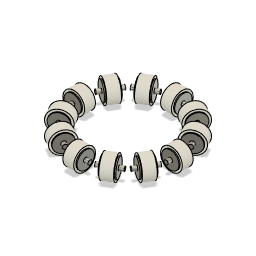
サイドホイール (Autodesk Fusion 360 design; units mm, degrees)
Autodesk Fusion 360 part; units mm, degrees
(part 1 of 3)
sketch "スケッチ1" plane through (0, 0.2306, 0) normal (0, 1, 0) x (-1, 0, 0)
  circle A0 centre (0.8985, -52.106) radius 15.5
  circle A1 centre (-6.9391, -68.3808) radius 1.5
  circle A2 centre (15.0212, -40.8435) radius 1.5
  circle A3 centre (-16.7123, -56.1256) radius 1.5
  circle A4 centre (8.736, -68.3808) radius 1.5
  circle A5 centre (0.8985, -34.0424) radius 1.5
  circle A6 centre (-13.2243, -40.8435) radius 1.5
  circle A7 centre (18.5092, -56.1256) radius 1.5
  arc A8 (-27.629, -49.2874) -> (-27.8547, -48.9282) centre (-27.9215, -49.2206) ccw
  line L0 (-27.8547, -48.9282) -> (-28.4097, -48.8015)
  arc A9 (-28.4097, -48.8015) -> (-28.9994, -49.6325) centre (-28.0028, -49.7149) ccw
  arc A10 (-28.9994, -49.6325) -> (-28.9994, -54.5796) centre (0.8985, -52.106) ccw
  arc A11 (-28.9994, -54.5796) -> (-28.4097, -55.4106) centre (-28.0028, -54.4971) ccw
  line L1 (-28.4097, -55.4106) -> (-27.8547, -55.2839)
  arc A12 (-27.8547, -55.2839) -> (-27.629, -54.9246) centre (-27.9215, -54.9914) ccw
  line L2 (-27.629, -54.9246) -> (-27.8404, -53.9985)
  arc A13 (-27.088, -52.801) -> (-27.8404, -53.9985) centre (-26.8654, -53.7759) ccw
  line L3 (-27.088, -52.801) -> (-26.308, -52.623)
  arc A14 (-25.1106, -53.3754) -> (-26.308, -52.623) centre (-26.0855, -53.5979) ccw
  line L4 (-25.1106, -53.3754) -> (-24.8992, -54.3016)
  arc A15 (-24.8992, -54.3016) -> (-24.5399, -54.5273) centre (-24.6067, -54.2348) ccw
  line L5 (-24.5399, -54.5273) -> (-20.6402, -53.6372)
  arc A16 (-19.4428, -54.3896) -> (-20.6402, -53.6372) centre (-20.4177, -54.6122) ccw
  line L6 (-19.4428, -54.3896) -> (-18.4192, -58.8743)
  arc A17 (-19.1716, -60.0718) -> (-18.4192, -58.8743) centre (-19.3941, -59.0968) ccw
  line L7 (-19.1716, -60.0718) -> (-22.9738, -60.9396)
  arc A18 (-22.9738, -60.9396) -> (-23.1995, -61.2988) centre (-22.9071, -61.2321) ccw
  line L8 (-23.1995, -61.2988) -> (-22.9881, -62.225)
  arc A19 (-23.7405, -63.4224) -> (-22.9881, -62.225) centre (-23.9631, -62.4475) ccw
  line L9 (-23.7405, -63.4224) -> (-24.618, -63.6227)
  arc A20 (-25.8154, -62.8703) -> (-24.618, -63.6227) centre (-24.8405, -62.6478) ccw
  line L10 (-25.8154, -62.8703) -> (-26.0268, -61.9441)
  arc A21 (-26.0268, -61.9441) -> (-26.3861, -61.7184) centre (-26.3193, -62.0109) ccw
  line L11 (-26.3861, -61.7184) -> (-26.9411, -61.8451)
  arc A22 (-26.9411, -61.8451) -> (-27.1118, -62.8496) centre (-26.1781, -62.4915) ccw
  arc A23 (-27.1118, -62.8496) -> (-24.9653, -67.3068) centre (0.8985, -52.106) ccw
  arc A24 (-24.9653, -67.3068) -> (-24.0735, -67.7997) centre (-24.1032, -66.8001) ccw
  line L12 (-24.0735, -67.7997) -> (-23.6284, -67.4447)
  arc A25 (-23.6284, -67.4447) -> (-23.5809, -67.0231) centre (-23.8155, -67.2102) ccw
  line L13 (-23.5809, -67.0231) -> (-24.1732, -66.2804)
  arc A26 (-24.0149, -64.8751) -> (-24.1732, -66.2804) centre (-23.3914, -65.6569) ccw
  line L14 (-24.0149, -64.8751) -> (-23.3894, -64.3763)
  arc A27 (-21.9841, -64.5346) -> (-23.3894, -64.3763) centre (-22.7659, -65.1581) ccw
  line L15 (-21.9841, -64.5346) -> (-21.3918, -65.2773)
  arc A28 (-21.3918, -65.2773) -> (-20.9702, -65.3248) centre (-21.1572, -65.0903) ccw
  line L16 (-20.9702, -65.3248) -> (-17.8429, -62.8309)
  arc A29 (-16.4375, -62.9892) -> (-17.8429, -62.8309) centre (-17.2194, -63.6127) ccw
  line L17 (-16.4375, -62.9892) -> (-13.5695, -66.5856)
  arc A30 (-13.7278, -67.991) -> (-13.5695, -66.5856) centre (-14.3513, -67.2091) ccw
  line L18 (-13.7278, -67.991) -> (-16.777, -70.4226)
  arc A31 (-16.777, -70.4226) -> (-16.8245, -70.8442) centre (-16.5899, -70.6571) ccw
  line L19 (-16.8245, -70.8442) -> (-16.2322, -71.5869)
  arc A32 (-16.3905, -72.9922) -> (-16.2322, -71.5869) centre (-17.014, -72.2104) ccw
  line L20 (-16.3905, -72.9922) -> (-17.0942, -73.5534)
  arc A33 (-18.4995, -73.395) -> (-17.0942, -73.5534) centre (-17.7176, -72.7715) ccw
  line L21 (-18.4995, -73.395) -> (-19.0918, -72.6523)
  arc A34 (-19.0918, -72.6523) -> (-19.5134, -72.6048) centre (-19.3263, -72.8393) ccw
  line L22 (-19.5134, -72.6048) -> (-19.9585, -72.9598)
  arc A35 (-19.9585, -72.9598) -> (-19.6764, -73.9389) centre (-18.9906, -73.2111) ccw
  arc A36 (-19.6764, -73.9389) -> (-15.8087, -77.0233) centre (0.8985, -52.106) ccw
  arc A37 (-15.8087, -77.0233) -> (-14.7913, -77.0804) centre (-15.2517, -76.1928) ccw
  line L23 (-14.7913, -77.0804) -> (-14.5443, -76.5675)
  arc A38 (-14.5443, -76.5675) -> (-14.6844, -76.1671) centre (-14.8146, -76.4374) ccw
  line L24 (-14.6844, -76.1671) -> (-15.5403, -75.7549)
  arc A39 (-16.0074, -74.42) -> (-15.5403, -75.7549) centre (-15.1065, -74.8539) ccw
  line L25 (-16.0074, -74.42) -> (-15.6603, -73.6992)
  arc A40 (-14.3255, -73.2322) -> (-15.6603, -73.6992) centre (-14.7593, -74.1331) ccw
  line L26 (-14.3255, -73.2322) -> (-13.4695, -73.6443)
  arc A41 (-13.4695, -73.6443) -> (-13.0691, -73.5042) centre (-13.3394, -73.3741) ccw
  line L27 (-13.0691, -73.5042) -> (-11.3335, -69.9003)
  arc A42 (-9.9987, -69.4333) -> (-11.3335, -69.9003) centre (-10.4326, -70.3342) ccw
  line L28 (-9.9987, -69.4333) -> (-5.8542, -71.4291)
  arc A43 (-5.3872, -72.764) -> (-5.8542, -71.4291) centre (-6.2881, -72.3301) ccw
  line L29 (-5.3872, -72.764) -> (-7.0793, -76.2778)
  arc A44 (-7.0793, -76.2778) -> (-6.9392, -76.6782) centre (-6.809, -76.4079) ccw
  line L30 (-6.9392, -76.6782) -> (-6.0833, -77.0904)
  arc A45 (-5.6162, -78.4253) -> (-6.0833, -77.0904) centre (-6.5171, -77.9914) ccw
  line L31 (-5.6162, -78.4253) -> (-6.0067, -79.2361)
  arc A46 (-7.3415, -79.7032) -> (-6.0067, -79.2361) centre (-6.9076, -78.8022) ccw
  line L32 (-7.3415, -79.7032) -> (-8.1974, -79.291)
  arc A47 (-8.1974, -79.291) -> (-8.5979, -79.4312) centre (-8.3276, -79.5613) ccw
  line L33 (-8.5979, -79.4312) -> (-8.8449, -79.9441)
  arc A48 (-8.8449, -79.9441) -> (-8.1659, -80.7039) centre (-7.8638, -79.7506) ccw
  arc A49 (-8.1659, -80.7039) -> (-3.3429, -81.8047) centre (0.8985, -52.106) ccw
  arc A50 (-3.3429, -81.8047) -> (-2.4015, -81.4147) centre (-3.2015, -80.8147) ccw
  line L34 (-2.4015, -81.4147) -> (-2.4015, -80.8454)
  arc A51 (-2.4015, -80.8454) -> (-2.7015, -80.5454) centre (-2.7015, -80.8454) ccw
  line L35 (-2.7015, -80.5454) -> (-3.6515, -80.5454)
  arc A52 (-4.6515, -79.5454) -> (-3.6515, -80.5454) centre (-3.6515, -79.5454) ccw
  line L36 (-4.6515, -79.5454) -> (-4.6515, -78.7454)
  arc A53 (-3.6515, -77.7454) -> (-4.6515, -78.7454) centre (-3.6515, -78.7454) ccw
  line L37 (-3.6515, -77.7454) -> (-2.7015, -77.7454)
  arc A54 (-2.7015, -77.7454) -> (-2.4015, -77.4454) centre (-2.7015, -77.4454) ccw
  line L38 (-2.4015, -77.4454) -> (-2.4015, -73.4454)
  arc A55 (-1.4015, -72.4454) -> (-2.4015, -73.4454) centre (-1.4015, -73.4454) ccw
  line L39 (-1.4015, -72.4454) -> (3.1985, -72.4454)
  arc A56 (4.1985, -73.4454) -> (3.1985, -72.4454) centre (3.1985, -73.4454) ccw
  line L40 (4.1985, -73.4454) -> (4.1985, -77.3454)
  arc A57 (4.1985, -77.3454) -> (4.4985, -77.6454) centre (4.4985, -77.3454) ccw
  line L41 (4.4985, -77.6454) -> (5.4485, -77.6454)
  arc A58 (6.4485, -78.6454) -> (5.4485, -77.6454) centre (5.4485, -78.6454) ccw
  line L42 (6.4485, -78.6454) -> (6.4485, -79.5454)
  arc A59 (5.4485, -80.5454) -> (6.4485, -79.5454) centre (5.4485, -79.5454) ccw
  line L43 (5.4485, -80.5454) -> (4.4985, -80.5454)
  arc A60 (4.4985, -80.5454) -> (4.1985, -80.8454) centre (4.4985, -80.8454) ccw
  line L44 (4.1985, -80.8454) -> (4.1985, -81.4147)
  arc A61 (4.1985, -81.4147) -> (5.1398, -81.8047) centre (4.9985, -80.8147) ccw
  arc A62 (5.1398, -81.8047) -> (9.9629, -80.7039) centre (0.8985, -52.106) ccw
  arc A63 (9.9629, -80.7039) -> (10.6418, -79.9441) centre (9.6607, -79.7506) ccw
  line L45 (10.6418, -79.9441) -> (10.3948, -79.4312)
  arc A64 (10.3948, -79.4312) -> (9.9944, -79.291) centre (10.1245, -79.5613) ccw
  line L46 (9.9944, -79.291) -> (9.1385, -79.7032)
  arc A65 (7.8036, -79.2361) -> (9.1385, -79.7032) centre (8.7046, -78.8022) ccw
  line L47 (7.8036, -79.2361) -> (7.4565, -78.5154)
  arc A66 (7.9236, -77.1805) -> (7.4565, -78.5154) centre (8.3575, -78.0815) ccw
  line L48 (7.9236, -77.1805) -> (8.7795, -76.7683)
  arc A67 (8.7795, -76.7683) -> (8.9196, -76.3679) centre (8.6493, -76.498) ccw
  line L49 (8.9196, -76.3679) -> (7.1841, -72.764)
  arc A68 (7.6512, -71.4291) -> (7.1841, -72.764) centre (8.0851, -72.3301) ccw
  line L50 (7.6512, -71.4291) -> (11.7956, -69.4333)
  arc A69 (13.1305, -69.9003) -> (11.7956, -69.4333) centre (12.2295, -70.3342) ccw
  line L51 (13.1305, -69.9003) -> (14.8226, -73.4141)
  arc A70 (14.8226, -73.4141) -> (15.2231, -73.5543) centre (15.0929, -73.284) ccw
  line L52 (15.2231, -73.5543) -> (16.079, -73.1421)
  arc A71 (17.4139, -73.6091) -> (16.079, -73.1421) centre (16.5129, -74.043) ccw
  line L53 (17.4139, -73.6091) -> (17.8044, -74.42)
  arc A72 (17.3373, -75.7549) -> (17.8044, -74.42) centre (16.9034, -74.8539) ccw
  line L54 (17.3373, -75.7549) -> (16.4814, -76.1671)
  arc A73 (16.4814, -76.1671) -> (16.3412, -76.5675) centre (16.6115, -76.4374) ccw
  line L55 (16.3412, -76.5675) -> (16.5882, -77.0804)
  arc A74 (16.5882, -77.0804) -> (17.6056, -77.0233) centre (17.0487, -76.1928) ccw
  arc A75 (17.6056, -77.0233) -> (21.3207, -74.0818) centre (0.8985, -52.106) ccw
  arc A76 (21.3207, -74.0818) -> (21.3281, -72.6237) centre (20.6399, -73.3492) ccw
  arc A77 (21.3281, -72.6237) -> (20.8871, -72.6543) centre (21.1217, -72.8414) ccw
  line L56 (20.8871, -72.6543) -> (20.2964, -73.395)
  arc A78 (18.8911, -73.5534) -> (20.2964, -73.395) centre (19.5146, -72.7715) ccw
  line L57 (18.8911, -73.5534) -> (18.2656, -73.0546)
  arc A79 (18.1073, -71.6493) -> (18.2656, -73.0546) centre (18.8891, -72.2728) ccw
  line L58 (18.1073, -71.6493) -> (18.6996, -70.9065)
  arc A80 (18.6996, -70.9065) -> (18.6521, -70.4849) centre (18.465, -70.7195) ccw
  line L59 (18.6521, -70.4849) -> (15.5248, -67.991)
  arc A81 (15.3664, -66.5856) -> (15.5248, -67.991) centre (16.1483, -67.2091) ccw
  line L60 (15.3664, -66.5856) -> (18.2345, -62.9892)
  arc A82 (19.6398, -62.8309) -> (18.2345, -62.9892) centre (19.0163, -63.6127) ccw
  line L61 (19.6398, -62.8309) -> (22.6889, -65.2625)
  arc A83 (22.6889, -65.2625) -> (23.1105, -65.215) centre (22.876, -65.0279) ccw
  line L62 (23.1105, -65.215) -> (23.7029, -64.4723)
  arc A84 (25.1082, -64.3139) -> (23.7029, -64.4723) centre (24.4847, -65.0957) ccw
  line L63 (25.1082, -64.3139) -> (25.8118, -64.8751)
  arc A85 (25.9702, -66.2804) -> (25.8118, -64.8751) centre (25.1883, -65.6569) ccw
  line L64 (25.9702, -66.2804) -> (25.3795, -67.0211)
  arc A86 (25.3795, -67.0211) -> (25.4477, -67.4579) centre (25.614, -67.2081) ccw
  arc A87 (25.4477, -67.4579) -> (26.8676, -67.1262) centre (26.002, -66.6255) ccw
  arc A88 (26.8676, -67.1262) -> (28.9087, -62.8496) centre (0.8985, -52.106) ccw
  arc A89 (28.9087, -62.8496) -> (28.738, -61.8451) centre (27.9751, -62.4915) ccw
  line L65 (28.738, -61.8451) -> (28.183, -61.7184)
  arc A90 (28.183, -61.7184) -> (27.8238, -61.9441) centre (28.1162, -62.0109) ccw
  line L66 (27.8238, -61.9441) -> (27.6124, -62.8703)
  arc A91 (26.4149, -63.6227) -> (27.6124, -62.8703) centre (26.6374, -62.6478) ccw
  line L67 (26.4149, -63.6227) -> (25.635, -63.4447)
  arc A92 (24.8826, -62.2473) -> (25.635, -63.4447) centre (25.8575, -62.4698) ccw
  line L68 (24.8826, -62.2473) -> (25.094, -61.3211)
  arc A93 (25.094, -61.3211) -> (24.8682, -60.9618) centre (24.8015, -61.2543) ccw
  line L69 (24.8682, -60.9618) -> (20.9685, -60.0718)
  arc A94 (20.2161, -58.8743) -> (20.9685, -60.0718) centre (21.1911, -59.0968) ccw
  line L70 (20.2161, -58.8743) -> (21.2397, -54.3896)
  arc A95 (22.4372, -53.6372) -> (21.2397, -54.3896) centre (22.2146, -54.6122) ccw
  line L71 (22.4372, -53.6372) -> (26.2394, -54.5051)
  arc A96 (26.2394, -54.5051) -> (26.5986, -54.2793) centre (26.3061, -54.2126) ccw
  line L72 (26.5986, -54.2793) -> (26.81, -53.3532)
  arc A97 (28.0075, -52.6007) -> (26.81, -53.3532) centre (27.7849, -53.5757) ccw
  line L73 (28.0075, -52.6007) -> (28.8849, -52.801)
  arc A98 (29.6373, -53.9985) -> (28.8849, -52.801) centre (28.6624, -53.7759) ccw
  line L74 (29.6373, -53.9985) -> (29.4259, -54.9246)
  arc A99 (29.4259, -54.9246) -> (29.6516, -55.2839) centre (29.7184, -54.9914) ccw
  line L75 (29.6516, -55.2839) -> (30.2067, -55.4106)
  arc A100 (30.2067, -55.4106) -> (30.7963, -54.5796) centre (29.7997, -54.4971) ccw
  arc A101 (30.7963, -54.5796) -> (30.7963, -49.6325) centre (0.8985, -52.106) ccw
  arc A102 (30.7963, -49.6325) -> (30.2067, -48.8015) centre (29.7997, -49.7149) ccw
  line L76 (30.2067, -48.8015) -> (29.6516, -48.9282)
  arc A103 (29.6516, -48.9282) -> (29.4259, -49.2874) centre (29.7184, -49.2206) ccw
  line L77 (29.4259, -49.2874) -> (29.6373, -50.2136)
  arc A104 (28.8849, -51.411) -> (29.6373, -50.2136) centre (28.6624, -50.4361) ccw
  line L78 (28.8849, -51.411) -> (28.105, -51.5891)
  arc A105 (26.9075, -50.8366) -> (28.105, -51.5891) centre (27.8824, -50.6141) ccw
  line L79 (26.9075, -50.8366) -> (26.6961, -49.9105)
  arc A106 (26.6961, -49.9105) -> (26.3369, -49.6847) centre (26.4036, -49.9772) ccw
  line L80 (26.3369, -49.6847) -> (22.4372, -50.5748)
  arc A107 (21.2397, -49.8224) -> (22.4372, -50.5748) centre (22.2146, -49.5999) ccw
  line L81 (21.2397, -49.8224) -> (20.2161, -45.3377)
  arc A108 (20.9685, -44.1403) -> (20.2161, -45.3377) centre (21.1911, -45.1152) ccw
  line L82 (20.9685, -44.1403) -> (24.7707, -43.2725)
  arc A109 (24.7707, -43.2725) -> (24.9965, -42.9132) centre (24.704, -42.98) ccw
  line L83 (24.9965, -42.9132) -> (24.7851, -41.9871)
  arc A110 (25.5375, -40.7896) -> (24.7851, -41.9871) centre (25.76, -41.7645) ccw
  line L84 (25.5375, -40.7896) -> (26.4149, -40.5893)
  arc A111 (27.6124, -41.3417) -> (26.4149, -40.5893) centre (26.6374, -41.5643) ccw
  line L85 (27.6124, -41.3417) -> (27.8238, -42.2679)
  arc A112 (27.8238, -42.2679) -> (28.183, -42.4936) centre (28.1162, -42.2012) ccw
  line L86 (28.183, -42.4936) -> (28.738, -42.367)
  arc A113 (28.738, -42.367) -> (28.9087, -41.3624) centre (27.9751, -41.7205) ccw
  arc A114 (28.9087, -41.3624) -> (26.7623, -36.9053) centre (0.8985, -52.106) ccw
  arc A115 (26.7623, -36.9053) -> (25.8705, -36.4124) centre (25.9001, -37.4119) ccw
  line L87 (25.8705, -36.4124) -> (25.4254, -36.7673)
  arc A116 (25.4254, -36.7673) -> (25.3779, -37.1889) centre (25.6124, -37.0019) ccw
  line L88 (25.3779, -37.1889) -> (25.9702, -37.9317)
  arc A117 (25.8118, -39.337) -> (25.9702, -37.9317) centre (25.1883, -38.5552) ccw
  line L89 (25.8118, -39.337) -> (25.1864, -39.8358)
  arc A118 (23.781, -39.6775) -> (25.1864, -39.8358) centre (24.5629, -39.054) ccw
  line L90 (23.781, -39.6775) -> (23.1887, -38.9347)
  arc A119 (23.1887, -38.9347) -> (22.7671, -38.8872) centre (22.9542, -39.1218) ccw
  line L91 (22.7671, -38.8872) -> (19.6398, -41.3812)
  arc A120 (18.2345, -41.2228) -> (19.6398, -41.3812) centre (19.0163, -40.5993) ccw
  line L92 (18.2345, -41.2228) -> (15.3664, -37.6264)
  arc A121 (15.5248, -36.2211) -> (15.3664, -37.6264) centre (16.1483, -37.0029) ccw
  line L93 (15.5248, -36.2211) -> (18.5739, -33.7895)
  arc A122 (18.5739, -33.7895) -> (18.6214, -33.3679) centre (18.3869, -33.5549) ccw
  line L94 (18.6214, -33.3679) -> (18.0291, -32.6251)
  arc A123 (18.1874, -31.2198) -> (18.0291, -32.6251) centre (18.8109, -32.0016) ccw
  line L95 (18.1874, -31.2198) -> (18.8911, -30.6587)
  arc A124 (20.2964, -30.817) -> (18.8911, -30.6587) centre (19.5146, -31.4405) ccw
  line L96 (20.2964, -30.817) -> (20.8887, -31.5598)
  arc A125 (20.8887, -31.5598) -> (21.3103, -31.6073) centre (21.1233, -31.3727) ccw
  line L97 (21.3103, -31.6073) -> (21.7554, -31.2523)
  arc A126 (21.7554, -31.2523) -> (21.4734, -30.2732) centre (20.7875, -31.0009) ccw
  arc A127 (21.4734, -30.2732) -> (17.6056, -27.1887) centre (0.8985, -52.106) ccw
  arc A128 (17.6056, -27.1887) -> (16.5882, -27.1316) centre (17.0487, -28.0193) ccw
  line L98 (16.5882, -27.1316) -> (16.3412, -27.6445)
  arc A129 (16.3412, -27.6445) -> (16.4814, -28.045) centre (16.6115, -27.7747) ccw
  line L99 (16.4814, -28.045) -> (17.3373, -28.4572)
  arc A130 (17.8044, -29.792) -> (17.3373, -28.4572) centre (16.9034, -29.3581) ccw
  line L100 (17.8044, -29.792) -> (17.4572, -30.5128)
  arc A131 (16.1224, -30.9799) -> (17.4572, -30.5128) centre (16.5563, -30.0789) ccw
  line L101 (16.1224, -30.9799) -> (15.2665, -30.5677)
  arc A132 (15.2665, -30.5677) -> (14.866, -30.7078) centre (15.1363, -30.838) ccw
  line L102 (14.866, -30.7078) -> (13.1305, -34.3117)
  arc A133 (11.7956, -34.7788) -> (13.1305, -34.3117) centre (12.2295, -33.8778) ccw
  line L103 (11.7956, -34.7788) -> (7.6512, -32.7829)
  arc A134 (7.1841, -31.4481) -> (7.6512, -32.7829) centre (8.0851, -31.882) ccw
  line L104 (7.1841, -31.4481) -> (8.8762, -27.9343)
  arc A135 (8.8762, -27.9343) -> (8.7361, -27.5338) centre (8.6059, -27.8041) ccw
  line L105 (8.7361, -27.5338) -> (7.8802, -27.1216)
  arc A136 (7.4131, -25.7868) -> (7.8802, -27.1216) centre (8.3141, -26.2207) ccw
  line L106 (7.4131, -25.7868) -> (7.8036, -24.9759)
  arc A137 (9.1385, -24.5088) -> (7.8036, -24.9759) centre (8.7046, -25.4098) ccw
  line L107 (9.1385, -24.5088) -> (9.9944, -24.921)
  arc A138 (9.9944, -24.921) -> (10.3948, -24.7809) centre (10.1245, -24.6507) ccw
  line L108 (10.3948, -24.7809) -> (10.6418, -24.268)
  arc A139 (10.6418, -24.268) -> (9.9629, -23.5082) centre (9.6607, -24.4614) ccw
  arc A140 (9.9629, -23.5082) -> (5.1398, -22.4074) centre (0.8985, -52.106) ccw
  arc A141 (5.1398, -22.4074) -> (4.1985, -22.7973) centre (4.9985, -23.3973) ccw
  line L109 (4.1985, -22.7973) -> (4.1985, -23.3666)
  arc A142 (4.1985, -23.3666) -> (4.4985, -23.6666) centre (4.4985, -23.3666) ccw
  line L110 (4.4985, -23.6666) -> (5.4485, -23.6666)
  arc A143 (6.4485, -24.6666) -> (5.4485, -23.6666) centre (5.4485, -24.6666) ccw
  line L111 (6.4485, -24.6666) -> (6.4485, -25.4666)
  arc A144 (5.4485, -26.4666) -> (6.4485, -25.4666) centre (5.4485, -25.4666) ccw
  line L112 (5.4485, -26.4666) -> (4.4985, -26.4666)
  arc A145 (4.4985, -26.4666) -> (4.1985, -26.7666) centre (4.4985, -26.7666) ccw
  line L113 (4.1985, -26.7666) -> (4.1985, -30.7666)
  arc A146 (3.1985, -31.7666) -> (4.1985, -30.7666) centre (3.1985, -30.7666) ccw
  line L114 (3.1985, -31.7666) -> (-1.4015, -31.7666)
  arc A147 (-2.4015, -30.7666) -> (-1.4015, -31.7666) centre (-1.4015, -30.7666) ccw
  line L115 (-2.4015, -30.7666) -> (-2.4015, -26.8666)
  arc A148 (-2.4015, -26.8666) -> (-2.7015, -26.5666) centre (-2.7015, -26.8666) ccw
  line L116 (-2.7015, -26.5666) -> (-3.6515, -26.5666)
  arc A149 (-4.6515, -25.5666) -> (-3.6515, -26.5666) centre (-3.6515, -25.5666) ccw
  line L117 (-4.6515, -25.5666) -> (-4.6515, -24.6666)
  arc A150 (-3.6515, -23.6666) -> (-4.6515, -24.6666) centre (-3.6515, -24.6666) ccw
  line L118 (-3.6515, -23.6666) -> (-2.7015, -23.6666)
  arc A151 (-2.7015, -23.6666) -> (-2.4015, -23.3666) centre (-2.7015, -23.3666) ccw
  line L119 (-2.4015, -23.3666) -> (-2.4015, -22.7973)
  arc A152 (-2.4015, -22.7973) -> (-3.3429, -22.4074) centre (-3.2015, -23.3973) ccw
  arc A153 (-3.3429, -22.4074) -> (-8.1659, -23.5082) centre (0.8985, -52.106) ccw
  arc A154 (-8.1659, -23.5082) -> (-8.8449, -24.268) centre (-7.8638, -24.4614) ccw
  line L120 (-8.8449, -24.268) -> (-8.5979, -24.7809)
  arc A155 (-8.5979, -24.7809) -> (-8.1974, -24.921) centre (-8.3276, -24.6507) ccw
  line L121 (-8.1974, -24.921) -> (-7.3415, -24.5088)
  arc A156 (-6.0067, -24.9759) -> (-7.3415, -24.5088) centre (-6.9076, -25.4098) ccw
  line L122 (-6.0067, -24.9759) -> (-5.6596, -25.6967)
  arc A157 (-6.1266, -27.0316) -> (-5.6596, -25.6967) centre (-6.5605, -26.1306) ccw
  line L123 (-6.1266, -27.0316) -> (-6.9826, -27.4437)
  arc A158 (-6.9826, -27.4437) -> (-7.1227, -27.8442) centre (-6.8524, -27.714) ccw
  line L124 (-7.1227, -27.8442) -> (-5.3872, -31.4481)
  arc A159 (-5.8542, -32.7829) -> (-5.3872, -31.4481) centre (-6.2881, -31.882) ccw
  line L125 (-5.8542, -32.7829) -> (-9.9987, -34.7788)
  arc A160 (-11.3335, -34.3117) -> (-9.9987, -34.7788) centre (-10.4326, -33.8778) ccw
  line L126 (-11.3335, -34.3117) -> (-13.0257, -30.7979)
  arc A161 (-13.0257, -30.7979) -> (-13.4262, -30.6578) centre (-13.296, -30.9281) ccw
  line L127 (-13.4262, -30.6578) -> (-14.2821, -31.07)
  arc A162 (-15.6169, -30.6029) -> (-14.2821, -31.07) centre (-14.716, -30.169) ccw
  line L128 (-15.6169, -30.6029) -> (-16.0074, -29.792)
  arc A163 (-15.5403, -28.4572) -> (-16.0074, -29.792) centre (-15.1065, -29.3581) ccw
  line L129 (-15.5403, -28.4572) -> (-14.6844, -28.045)
  arc A164 (-14.6844, -28.045) -> (-14.5443, -27.6445) centre (-14.8146, -27.7747) ccw
  line L130 (-14.5443, -27.6445) -> (-14.7913, -27.1316)
  arc A165 (-14.7913, -27.1316) -> (-15.8087, -27.1887) centre (-15.2517, -28.0193) ccw
  arc A166 (-15.8087, -27.1887) -> (-19.6764, -30.2732) centre (0.8985, -52.106) ccw
  arc A167 (-19.6764, -30.2732) -> (-19.9585, -31.2523) centre (-18.9906, -31.0009) ccw
  line L131 (-19.9585, -31.2523) -> (-19.5134, -31.6073)
  arc A168 (-19.5134, -31.6073) -> (-19.0918, -31.5598) centre (-19.3263, -31.3727) ccw
  line L132 (-19.0918, -31.5598) -> (-18.4995, -30.817)
  arc A169 (-17.0942, -30.6587) -> (-18.4995, -30.817) centre (-17.7176, -31.4405) ccw
  line L133 (-17.0942, -30.6587) -> (-16.4687, -31.1575)
  arc A170 (-16.3103, -32.5628) -> (-16.4687, -31.1575) centre (-17.0922, -31.9393) ccw
  line L134 (-16.3103, -32.5628) -> (-16.9027, -33.3055)
  arc A171 (-16.9027, -33.3055) -> (-16.8552, -33.7271) centre (-16.6681, -33.4926) ccw
  line L135 (-16.8552, -33.7271) -> (-13.7278, -36.2211)
  arc A172 (-13.5695, -37.6264) -> (-13.7278, -36.2211) centre (-14.3513, -37.0029) ccw
  line L136 (-13.5695, -37.6264) -> (-16.4375, -41.2228)
  arc A173 (-17.8429, -41.3812) -> (-16.4375, -41.2228) centre (-17.2194, -40.5993) ccw
  line L137 (-17.8429, -41.3812) -> (-20.892, -38.9496)
  arc A174 (-20.892, -38.9496) -> (-21.3136, -38.9971) centre (-21.0791, -39.1841) ccw
  line L138 (-21.3136, -38.9971) -> (-21.9059, -39.7398)
  arc A175 (-23.3112, -39.8981) -> (-21.9059, -39.7398) centre (-22.6878, -39.1163) ccw
  line L139 (-23.3112, -39.8981) -> (-24.0149, -39.337)
  arc A176 (-24.1732, -37.9317) -> (-24.0149, -39.337) centre (-23.3914, -38.5552) ccw
  line L140 (-24.1732, -37.9317) -> (-23.5809, -37.1889)
  arc A177 (-23.5809, -37.1889) -> (-23.6284, -36.7673) centre (-23.8155, -37.0019) ccw
  line L141 (-23.6284, -36.7673) -> (-24.0735, -36.4124)
  arc A178 (-24.0735, -36.4124) -> (-24.9653, -36.9053) centre (-24.1032, -37.4119) ccw
  arc A179 (-24.9653, -36.9053) -> (-27.1118, -41.3624) centre (0.8985, -52.106) ccw
  arc A180 (-27.1118, -41.3624) -> (-26.9411, -42.367) centre (-26.1781, -41.7205) ccw
  line L142 (-26.9411, -42.367) -> (-26.3861, -42.4936)
  arc A181 (-26.3861, -42.4936) -> (-26.0268, -42.2679) centre (-26.3193, -42.2012) ccw
  line L143 (-26.0268, -42.2679) -> (-25.8154, -41.3417)
  arc A182 (-24.618, -40.5893) -> (-25.8154, -41.3417) centre (-24.8405, -41.5643) ccw
  line L144 (-24.618, -40.5893) -> (-23.838, -40.7674)
  arc A183 (-23.0856, -41.9648) -> (-23.838, -40.7674) centre (-24.0606, -41.7423) ccw
  line L145 (-23.0856, -41.9648) -> (-23.297, -42.891)
  arc A184 (-23.297, -42.891) -> (-23.0713, -43.2502) centre (-23.0045, -42.9577) ccw
  line L146 (-23.0713, -43.2502) -> (-19.1716, -44.1403)
  arc A185 (-18.4192, -45.3377) -> (-19.1716, -44.1403) centre (-19.3941, -45.1152) ccw
  line L147 (-18.4192, -45.3377) -> (-19.4428, -49.8224)
  arc A186 (-20.6402, -50.5748) -> (-19.4428, -49.8224) centre (-20.4177, -49.5999) ccw
  line L148 (-20.6402, -50.5748) -> (-24.4424, -49.707)
  arc A187 (-24.4424, -49.707) -> (-24.8017, -49.9327) centre (-24.5092, -49.9995) ccw
  line L149 (-24.8017, -49.9327) -> (-25.0131, -50.8589)
  arc A188 (-26.2105, -51.6113) -> (-25.0131, -50.8589) centre (-25.988, -50.6364) ccw
  line L150 (-26.2105, -51.6113) -> (-27.088, -51.411)
  arc A189 (-27.8404, -50.2136) -> (-27.088, -51.411) centre (-26.8654, -50.4361) ccw
  line L151 (-27.8404, -50.2136) -> (-27.629, -49.2874)
  line L152 (4.1985, -80.8454) -> (4.1985, -80.8)
  line L153 (4.1985, -81.4147) -> (4.1985, -81.9391)
  line L154 (-2.4015, -81.4147) -> (-2.4015, -81.9846)
  line L155 (4.1985, -81.4147) -> (4.1985, -80.5454)
  line L156 (4.4985, -80.5454) -> (4.1985, -80.5454)
  line L157 (4.4985, -80.5454) -> (6.4485, -80.5454)
  line L158 (6.4485, -79.5454) -> (6.4485, -80.5454)
  line L159 (6.4485, -79.5454) -> (6.4485, -77.6454)
  line L160 (5.4485, -77.6454) -> (6.4485, -77.6454)
  line L161 (5.4485, -77.6454) -> (4.1985, -77.6454)
  line L162 (4.1985, -77.3454) -> (4.1985, -77.6454)
  line L163 (4.1985, -77.3454) -> (4.1985, -72.4454)
  line L164 (3.1985, -72.4454) -> (4.1985, -72.4454)
  line L165 (3.1985, -72.4454) -> (-2.4015, -72.4454)
  line L166 (-2.4015, -73.4454) -> (-2.4015, -72.4454)
  line L167 (-2.4015, -73.4454) -> (-2.4015, -77.7454)
  line L168 (-3.1765, -77.7454) -> (-2.4015, -77.7454)
  line L169 (-3.1765, -77.7454) -> (-4.6515, -77.7454)
  line L170 (-4.6515, -78.7454) -> (-4.6515, -77.7454)
  line L171 (-4.6515, -78.7454) -> (-4.6515, -80.5454)
  line L172 (-3.6515, -80.5454) -> (-4.6515, -80.5454)
  line L173 (-3.6515, -80.5454) -> (-2.4015, -80.5454)
  line L174 (-2.4015, -81.4147) -> (-2.4015, -80.5454)
  line L175 (5.55, -232.8464) -> (5.55, -231.9464)
  line L176 (3.6, -233.8464) -> (4.55, -233.8464)
  line L177 (-3.6, -233.8464) -> (-4.55, -233.8464)
  line L178 (-5.55, -232.0464) -> (-5.55, -232.8464)
  line L179 (-3.3, -234.1464) -> (-3.3, -234.7095)
  line L180 (-3.3, -226.7464) -> (-3.3, -230.7464)
  line L181 (3.3, -234.1464) -> (3.3, -234.7095)
  line L182 (-3.6, -231.0464) -> (-4.55, -231.0464)
  line L183 (4.55, -230.9464) -> (3.6, -230.9464)
  line L184 (2.3, -225.7464) -> (-2.3, -225.7464)
  line L185 (3.3, -230.6464) -> (3.3, -226.7464)
  arc A190 (4.55, -233.8464) -> (5.55, -232.8464) centre (4.55, -232.8464) ccw
  arc A191 (5.55, -231.9464) -> (4.55, -230.9464) centre (4.55, -231.9464) ccw
  arc A192 (-5.55, -232.8464) -> (-4.55, -233.8464) centre (-4.55, -232.8464) ccw
  arc A193 (-4.55, -231.0464) -> (-5.55, -232.0464) centre (-4.55, -232.0464) ccw
  arc A194 (3.3, -226.7464) -> (2.3, -225.7464) centre (2.3, -226.7464) ccw
  arc A195 (-2.3, -225.7464) -> (-3.3, -226.7464) centre (-2.3, -226.7464) ccw
  arc A196 (3.3, -230.6464) -> (3.6, -230.9464) centre (3.6, -230.6464) ccw
  arc A197 (3.6, -233.8464) -> (3.3, -234.1464) centre (3.6, -234.1464) ccw
  arc A198 (-3.3, -234.1464) -> (-3.6, -233.8464) centre (-3.6, -234.1464) ccw
  arc A199 (-3.6, -231.0464) -> (-3.3, -230.7464) centre (-3.6, -230.7464) ccw
  arc A200 (3.3, -234.7095) -> (3.876, -235.2037) centre (3.8, -234.7095) ccw
  arc A201 (-3.876, -235.2037) -> (-3.3, -234.7095) centre (-3.8, -234.7095) ccw
  arc A202 (9.2153, -232.5614) -> (8.8055, -232.4516) centre (8.9555, -232.7114) ccw
  arc A203 (6.5828, -230.5018) -> (6.2168, -231.8678) centre (7.0828, -231.3678) ccw
  arc A204 (5.8814, -224.7868) -> (5.5153, -226.1528) centre (6.3814, -225.6528) ccw
  arc A205 (11.2311, -222.8528) -> (9.8651, -222.4868) centre (10.3651, -223.3528) ccw
  line L186 (14.9311, -229.2614) -> (15.2126, -229.7491)
  line L187 (8.8055, -232.4516) -> (7.9828, -232.9266)
  arc A206 (9.2451, -233.765) -> (9.4969, -233.0491) centre (9.0639, -233.2991) ccw
  line L188 (6.2168, -231.8678) -> (6.6168, -232.5606)
  line L189 (7.4055, -230.0268) -> (6.5828, -230.5018)
  line L190 (9.2153, -232.5614) -> (9.4969, -233.0491)
  line L191 (13.1811, -226.2303) -> (11.2311, -222.8528)
  arc A207 (6.6168, -232.5606) -> (7.9828, -232.9266) centre (7.4828, -232.0606) ccw
  line L192 (9.8651, -222.4868) -> (5.8814, -224.7868)
  arc A208 (7.4055, -230.0268) -> (7.5153, -229.6169) centre (7.2555, -229.7669) ccw
  line L193 (5.5153, -226.1528) -> (7.5153, -229.6169)
  arc A209 (15.2126, -229.7491) -> (15.9586, -229.889) centre (15.6457, -229.4991) ccw
  arc A210 (15.7797, -226.2312) -> (14.4136, -225.8651) centre (14.9136, -226.7312) ccw
  line L194 (15.0409, -228.8516) -> (15.8636, -228.3766)
  line L195 (16.2297, -227.0106) -> (15.7797, -226.2312)
  line L196 (14.4136, -225.8651) -> (13.5909, -226.3401)
  arc A211 (15.0409, -228.8516) -> (14.9311, -229.2614) centre (15.1909, -229.1114) ccw
  arc A212 (13.1811, -226.2303) -> (13.5909, -226.3401) centre (13.4409, -226.0803) ccw
  arc A213 (15.8636, -228.3766) -> (16.2297, -227.0106) centre (15.3636, -227.5106) ccw
  arc A214 (19.2614, -224.9311) -> (18.8516, -225.0409) centre (19.1114, -225.1909) ccw
  arc A215 (15.9517, -224.4636) -> (16.3178, -225.8297) centre (16.8178, -224.9636) ccw
  arc A216 (12.4868, -219.8651) -> (12.8528, -221.2311) centre (13.3528, -220.3651) ccw
  arc A217 (16.1528, -215.5153) -> (14.7868, -215.8814) centre (15.6528, -216.3814) ccw
  line L197 (22.5614, -219.2153) -> (23.0491, -219.4969)
  line L198 (18.8516, -225.0409) -> (18.3766, -225.8636)
  arc A218 (19.889, -225.9586) -> (19.7491, -225.2126) centre (19.4991, -225.6457) ccw
  line L199 (16.3178, -225.8297) -> (17.0106, -226.2297)
  line L200 (16.4267, -223.6409) -> (15.9517, -224.4636)
  line L201 (19.2614, -224.9311) -> (19.7491, -225.2126)
  line L202 (19.5303, -217.4653) -> (16.1528, -215.5153)
  arc A219 (17.0106, -226.2297) -> (18.3766, -225.8636) centre (17.5106, -225.3636) ccw
  line L203 (14.7868, -215.8814) -> (12.4868, -219.8651)
  arc A220 (16.4267, -223.6409) -> (16.3169, -223.2311) centre (16.1669, -223.4909) ccw
  line L204 (12.8528, -221.2311) -> (16.3169, -223.2311)
  arc A221 (23.0491, -219.4969) -> (23.765, -219.2451) centre (23.2991, -219.0639) ccw
  arc A222 (21.7812, -216.1668) -> (20.4151, -216.5328) centre (21.2812, -217.0328) ccw
  line L205 (22.4516, -218.8055) -> (22.9266, -217.9828)
  line L206 (22.5606, -216.6168) -> (21.7812, -216.1668)
  line L207 (20.4151, -216.5328) -> (19.9401, -217.3555)
  arc A223 (22.4516, -218.8055) -> (22.5614, -219.2153) centre (22.7114, -218.9555) ccw
  arc A224 (19.5303, -217.4653) -> (19.9401, -217.3555) centre (19.6803, -217.2055) ccw
  arc A225 (22.9266, -217.9828) -> (22.5606, -216.6168) centre (22.0606, -217.4828) ccw
  arc A226 (24.1464, -213.3) -> (23.8464, -213.6) centre (24.1464, -213.6) ccw
  arc A227 (21.0464, -214.55) -> (22.0464, -215.55) centre (22.0464, -214.55) ccw
  arc A228 (15.7464, -212.3) -> (16.7464, -213.3) centre (16.7464, -212.3) ccw
  arc A229 (16.7464, -206.7) -> (15.7464, -207.7) centre (16.7464, -207.7) ccw
  line L208 (24.1464, -206.7) -> (24.7095, -206.7)
  line L209 (23.8464, -213.6) -> (23.8464, -214.55)
  arc A230 (25.2037, -213.876) -> (24.7095, -213.3) centre (24.7095, -213.8) ccw
  line L210 (22.0464, -215.55) -> (22.8464, -215.55)
  line L211 (21.0464, -213.6) -> (21.0464, -214.55)
  line L212 (24.1464, -213.3) -> (24.7095, -213.3)
  line L213 (20.6464, -206.7) -> (16.7464, -206.7)
  arc A231 (22.8464, -215.55) -> (23.8464, -214.55) centre (22.8464, -214.55) ccw
  line L214 (15.7464, -207.7) -> (15.7464, -212.3)
  arc A232 (21.0464, -213.6) -> (20.7464, -213.3) centre (20.7464, -213.6) ccw
  line L215 (16.7464, -213.3) -> (20.7464, -213.3)
  arc A233 (24.7095, -206.7) -> (25.2037, -206.124) centre (24.7095, -206.2) ccw
  arc A234 (21.9464, -204.45) -> (20.9464, -205.45) centre (21.9464, -205.45) ccw
  line L216 (23.8464, -206.4) -> (23.8464, -205.45)
  line L217 (22.8464, -204.45) -> (21.9464, -204.45)
  line L218 (20.9464, -205.45) -> (20.9464, -206.4)
  arc A235 (23.8464, -206.4) -> (24.1464, -206.7) centre (24.1464, -206.4) ccw
  arc A236 (20.6464, -206.7) -> (20.9464, -206.4) centre (20.6464, -206.4) ccw
  arc A237 (23.8464, -205.45) -> (22.8464, -204.45) centre (22.8464, -205.45) ccw
  arc A238 (22.5614, -200.7847) -> (22.4516, -201.1945) centre (22.7114, -201.0445) ccw
  arc A239 (20.5017, -203.4172) -> (21.8678, -203.7832) centre (21.3678, -202.9172) ccw
  arc A240 (14.7868, -204.1186) -> (16.1528, -204.4847) centre (15.6528, -203.6186) ccw
  arc A241 (12.8528, -198.7689) -> (12.4868, -200.1349) centre (13.3528, -199.6349) ccw
  line L219 (19.2614, -195.0689) -> (19.7491, -194.7874)
  line L220 (22.4516, -201.1945) -> (22.9266, -202.0172)
  arc A242 (23.765, -200.7549) -> (23.0491, -200.5031) centre (23.2991, -200.9361) ccw
  line L221 (21.8678, -203.7832) -> (22.5606, -203.3832)
  line L222 (20.0267, -202.5945) -> (20.5017, -203.4172)
  line L223 (22.5614, -200.7847) -> (23.0491, -200.5031)
  line L224 (16.2303, -196.8189) -> (12.8528, -198.7689)
  arc A243 (22.5606, -203.3832) -> (22.9266, -202.0172) centre (22.0606, -202.5172) ccw
  line L225 (12.4868, -200.1349) -> (14.7868, -204.1186)
  arc A244 (20.0267, -202.5945) -> (19.6169, -202.4847) centre (19.7669, -202.7445) ccw
  line L226 (16.1528, -204.4847) -> (19.6169, -202.4847)
  arc A245 (19.7491, -194.7874) -> (19.889, -194.0414) centre (19.4991, -194.3544) ccw
  arc A246 (16.2312, -194.2203) -> (15.8651, -195.5864) centre (16.7312, -195.0864) ccw
  line L227 (18.8516, -194.9591) -> (18.3766, -194.1364)
  line L228 (17.0106, -193.7703) -> (16.2312, -194.2203)
  line L229 (15.8651, -195.5864) -> (16.3401, -196.4091)
  arc A247 (18.8516, -194.9591) -> (19.2614, -195.0689) centre (19.1114, -194.8091) ccw
  arc A248 (16.2303, -196.8189) -> (16.3401, -196.4091) centre (16.0803, -196.5591) ccw
  arc A249 (18.3766, -194.1364) -> (17.0106, -193.7703) centre (17.5106, -194.6364) ccw
  arc A250 (14.9311, -190.7386) -> (15.0409, -191.1484) centre (15.1909, -190.8886) ccw
  arc A251 (14.4636, -194.0483) -> (15.8297, -193.6822) centre (14.9636, -193.1822) ccw
  arc A252 (9.8651, -197.5132) -> (11.2311, -197.1472) centre (10.3651, -196.6472) ccw
  arc A253 (5.5153, -193.8472) -> (5.8814, -195.2132) centre (6.3814, -194.3472) ccw
  line L230 (9.2153, -187.4386) -> (9.4969, -186.9509)
  line L231 (15.0409, -191.1484) -> (15.8636, -191.6234)
  arc A254 (15.9586, -190.111) -> (15.2126, -190.2509) centre (15.6457, -190.5009) ccw
  line L232 (15.8297, -193.6822) -> (16.2297, -192.9894)
  line L233 (13.6409, -193.5733) -> (14.4636, -194.0483)
  line L234 (14.9311, -190.7386) -> (15.2126, -190.2509)
  line L235 (7.4653, -190.4697) -> (5.5153, -193.8472)
  arc A255 (16.2297, -192.9894) -> (15.8636, -191.6234) centre (15.3636, -192.4894) ccw
  line L236 (5.8814, -195.2132) -> (9.8651, -197.5132)
  arc A256 (13.6409, -193.5733) -> (13.2311, -193.6831) centre (13.4909, -193.8331) ccw
  line L237 (11.2311, -197.1472) -> (13.2311, -193.6831)
  arc A257 (9.4969, -186.9509) -> (9.2451, -186.235) centre (9.0639, -186.7009) ccw
  arc A258 (6.1668, -188.2188) -> (6.5328, -189.5849) centre (7.0328, -188.7188) ccw
  line L238 (8.8055, -187.5484) -> (7.9828, -187.0734)
  line L239 (6.6168, -187.4394) -> (6.1668, -188.2188)
  line L240 (6.5328, -189.5849) -> (7.3555, -190.0599)
  arc A259 (8.8055, -187.5484) -> (9.2153, -187.4386) centre (8.9555, -187.2886) ccw
  arc A260 (7.4653, -190.4697) -> (7.3555, -190.0599) centre (7.2055, -190.3197) ccw
  arc A261 (7.9828, -187.0734) -> (6.6168, -187.4394) centre (7.4828, -187.9394) ccw
  arc A262 (3.3, -185.8536) -> (3.6, -186.1536) centre (3.6, -185.8536) ccw
  arc A263 (4.55, -188.9536) -> (5.55, -187.9536) centre (4.55, -187.9536) ccw
  arc A264 (2.3, -194.2536) -> (3.3, -193.2536) centre (2.3, -193.2536) ccw
  arc A265 (-3.3, -193.2536) -> (-2.3, -194.2536) centre (-2.3, -193.2536) ccw
  line L241 (-3.3, -185.8536) -> (-3.3, -185.2905)
  line L242 (3.6, -186.1536) -> (4.55, -186.1536)
  arc A266 (3.876, -184.7963) -> (3.3, -185.2905) centre (3.8, -185.2905) ccw
  line L243 (5.55, -187.9536) -> (5.55, -187.1536)
  line L244 (3.6, -188.9536) -> (4.55, -188.9536)
  line L245 (3.3, -185.8536) -> (3.3, -185.2905)
  line L246 (-3.3, -189.3536) -> (-3.3, -193.2536)
  arc A267 (5.55, -187.1536) -> (4.55, -186.1536) centre (4.55, -187.1536) ccw
  line L247 (-2.3, -194.2536) -> (2.3, -194.2536)
  arc A268 (3.6, -188.9536) -> (3.3, -189.2536) centre (3.6, -189.2536) ccw
  line L248 (3.3, -193.2536) -> (3.3, -189.2536)
  arc A269 (-3.3, -185.2905) -> (-3.876, -184.7963) centre (-3.8, -185.2905) ccw
  arc A270 (-5.55, -188.0536) -> (-4.55, -189.0536) centre (-4.55, -188.0536) ccw
  line L249 (-3.6, -186.1536) -> (-4.55, -186.1536)
  line L250 (-5.55, -187.1536) -> (-5.55, -188.0536)
  line L251 (-4.55, -189.0536) -> (-3.6, -189.0536)
  arc A271 (-3.6, -186.1536) -> (-3.3, -185.8536) centre (-3.6, -185.8536) ccw
  arc A272 (-3.3, -189.3536) -> (-3.6, -189.0536) centre (-3.6, -189.3536) ccw
  arc A273 (-4.55, -186.1536) -> (-5.55, -187.1536) centre (-4.55, -187.1536) ccw
  arc A274 (-9.2153, -187.4386) -> (-8.8055, -187.5484) centre (-8.9555, -187.2886) ccw
  arc A275 (-6.5828, -189.4983) -> (-6.2168, -188.1322) centre (-7.0828, -188.6322) ccw
  arc A276 (-5.8814, -195.2132) -> (-5.5153, -193.8472) centre (-6.3814, -194.3472) ccw
  arc A277 (-11.2311, -197.1472) -> (-9.8651, -197.5132) centre (-10.3651, -196.6472) ccw
  line L252 (-14.9311, -190.7386) -> (-15.2126, -190.2509)
  line L253 (-8.8055, -187.5484) -> (-7.9828, -187.0734)
  arc A278 (-9.2451, -186.235) -> (-9.4969, -186.9509) centre (-9.0639, -186.7009) ccw
  line L254 (-6.2168, -188.1322) -> (-6.6168, -187.4394)
  line L255 (-7.4055, -189.9733) -> (-6.5828, -189.4983)
  line L256 (-9.2153, -187.4386) -> (-9.4969, -186.9509)
  line L257 (-13.1811, -193.7697) -> (-11.2311, -197.1472)
  arc A279 (-6.6168, -187.4394) -> (-7.9828, -187.0734) centre (-7.4828, -187.9394) ccw
  line L258 (-9.8651, -197.5132) -> (-5.8814, -195.2132)
  arc A280 (-7.4055, -189.9733) -> (-7.5153, -190.3831) centre (-7.2555, -190.2331) ccw
  line L259 (-5.5153, -193.8472) -> (-7.5153, -190.3831)
  arc A281 (-15.2126, -190.2509) -> (-15.9586, -190.111) centre (-15.6457, -190.5009) ccw
  arc A282 (-15.7797, -193.7688) -> (-14.4136, -194.1349) centre (-14.9136, -193.2688) ccw
  line L260 (-15.0409, -191.1484) -> (-15.8636, -191.6234)
  line L261 (-16.2297, -192.9894) -> (-15.7797, -193.7688)
  line L262 (-14.4136, -194.1349) -> (-13.5909, -193.6599)
  arc A283 (-15.0409, -191.1484) -> (-14.9311, -190.7386) centre (-15.1909, -190.8886) ccw
  arc A284 (-13.1811, -193.7697) -> (-13.5909, -193.6599) centre (-13.4409, -193.9197) ccw
  arc A285 (-15.8636, -191.6234) -> (-16.2297, -192.9894) centre (-15.3636, -192.4894) ccw
  arc A286 (-19.2614, -195.0689) -> (-18.8516, -194.9591) centre (-19.1114, -194.8091) ccw
  arc A287 (-15.9517, -195.5364) -> (-16.3178, -194.1703) centre (-16.8178, -195.0364) ccw
  arc A288 (-12.4868, -200.1349) -> (-12.8528, -198.7689) centre (-13.3528, -199.6349) ccw
  arc A289 (-16.1528, -204.4847) -> (-14.7868, -204.1186) centre (-15.6528, -203.6186) ccw
  line L263 (-22.5614, -200.7847) -> (-23.0491, -200.5031)
  line L264 (-18.8516, -194.9591) -> (-18.3766, -194.1364)
  arc A290 (-19.889, -194.0414) -> (-19.7491, -194.7874) centre (-19.4991, -194.3544) ccw
  line L265 (-16.3178, -194.1703) -> (-17.0106, -193.7703)
  line L266 (-16.4267, -196.3591) -> (-15.9517, -195.5364)
  line L267 (-19.2614, -195.0689) -> (-19.7491, -194.7874)
  line L268 (-19.5303, -202.5347) -> (-16.1528, -204.4847)
  arc A291 (-17.0106, -193.7703) -> (-18.3766, -194.1364) centre (-17.5106, -194.6364) ccw
  line L269 (-14.7868, -204.1186) -> (-12.4868, -200.1349)
  arc A292 (-16.4267, -196.3591) -> (-16.3169, -196.7689) centre (-16.1669, -196.5091) ccw
  line L270 (-12.8528, -198.7689) -> (-16.3169, -196.7689)
  arc A293 (-23.0491, -200.5031) -> (-23.765, -200.7549) centre (-23.2991, -200.9361) ccw
  arc A294 (-21.7812, -203.8332) -> (-20.4151, -203.4672) centre (-21.2812, -202.9672) ccw
  line L271 (-22.4516, -201.1945) -> (-22.9266, -202.0172)
  line L272 (-22.5606, -203.3832) -> (-21.7812, -203.8332)
  line L273 (-20.4151, -203.4672) -> (-19.9401, -202.6445)
  arc A295 (-22.4516, -201.1945) -> (-22.5614, -200.7847) centre (-22.7114, -201.0445) ccw
  arc A296 (-19.5303, -202.5347) -> (-19.9401, -202.6445) centre (-19.6803, -202.7945) ccw
  arc A297 (-22.9266, -202.0172) -> (-22.5606, -203.3832) centre (-22.0606, -202.5172) ccw
  arc A298 (-24.1464, -206.7) -> (-23.8464, -206.4) centre (-24.1464, -206.4) ccw
  arc A299 (-21.0464, -205.45) -> (-22.0464, -204.45) centre (-22.0464, -205.45) ccw
  arc A300 (-15.7464, -207.7) -> (-16.7464, -206.7) centre (-16.7464, -207.7) ccw
  arc A301 (-16.7464, -213.3) -> (-15.7464, -212.3) centre (-16.7464, -212.3) ccw
  line L274 (-24.1464, -213.3) -> (-24.7095, -213.3)
  line L275 (-23.8464, -206.4) -> (-23.8464, -205.45)
  arc A302 (-25.2037, -206.124) -> (-24.7095, -206.7) centre (-24.7095, -206.2) ccw
  line L276 (-22.0464, -204.45) -> (-22.8464, -204.45)
  line L277 (-21.0464, -206.4) -> (-21.0464, -205.45)
  line L278 (-24.1464, -206.7) -> (-24.7095, -206.7)
  line L279 (-20.6464, -213.3) -> (-16.7464, -213.3)
  arc A303 (-22.8464, -204.45) -> (-23.8464, -205.45) centre (-22.8464, -205.45) ccw
  line L280 (-15.7464, -212.3) -> (-15.7464, -207.7)
  arc A304 (-21.0464, -206.4) -> (-20.7464, -206.7) centre (-20.7464, -206.4) ccw
  line L281 (-16.7464, -206.7) -> (-20.7464, -206.7)
  arc A305 (-24.7095, -213.3) -> (-25.2037, -213.876) centre (-24.7095, -213.8) ccw
  arc A306 (-21.9464, -215.55) -> (-20.9464, -214.55) centre (-21.9464, -214.55) ccw
  line L282 (-23.8464, -213.6) -> (-23.8464, -214.55)
  line L283 (-22.8464, -215.55) -> (-21.9464, -215.55)
  line L284 (-20.9464, -214.55) -> (-20.9464, -213.6)
  arc A307 (-23.8464, -213.6) -> (-24.1464, -213.3) centre (-24.1464, -213.6) ccw
  arc A308 (-20.6464, -213.3) -> (-20.9464, -213.6) centre (-20.6464, -213.6) ccw
  arc A309 (-23.8464, -214.55) -> (-22.8464, -215.55) centre (-22.8464, -214.55) ccw
  arc A310 (-22.5614, -219.2153) -> (-22.4516, -218.8055) centre (-22.7114, -218.9555) ccw
  arc A311 (-20.5017, -216.5828) -> (-21.8678, -216.2168) centre (-21.3678, -217.0828) ccw
  arc A312 (-14.7868, -215.8814) -> (-16.1528, -215.5153) centre (-15.6528, -216.3814) ccw
  arc A313 (-12.8528, -221.2311) -> (-12.4868, -219.8651) centre (-13.3528, -220.3651) ccw
  line L285 (-19.2614, -224.9311) -> (-19.7491, -225.2126)
  line L286 (-22.4516, -218.8055) -> (-22.9266, -217.9828)
  arc A314 (-23.765, -219.2451) -> (-23.0491, -219.4969) centre (-23.2991, -219.0639) ccw
  line L287 (-21.8678, -216.2168) -> (-22.5606, -216.6168)
  line L288 (-20.0267, -217.4055) -> (-20.5017, -216.5828)
  line L289 (-22.5614, -219.2153) -> (-23.0491, -219.4969)
  line L290 (-16.2303, -223.1811) -> (-12.8528, -221.2311)
  arc A315 (-22.5606, -216.6168) -> (-22.9266, -217.9828) centre (-22.0606, -217.4828) ccw
  line L291 (-12.4868, -219.8651) -> (-14.7868, -215.8814)
  arc A316 (-20.0267, -217.4055) -> (-19.6169, -217.5153) centre (-19.7669, -217.2555) ccw
  line L292 (-16.1528, -215.5153) -> (-19.6169, -217.5153)
  arc A317 (-19.7491, -225.2126) -> (-19.889, -225.9586) centre (-19.4991, -225.6457) ccw
  arc A318 (-16.2312, -225.7797) -> (-15.8651, -224.4136) centre (-16.7312, -224.9136) ccw
  line L293 (-18.8516, -225.0409) -> (-18.3766, -225.8636)
  line L294 (-17.0106, -226.2297) -> (-16.2312, -225.7797)
  line L295 (-15.8651, -224.4136) -> (-16.3401, -223.5909)
  arc A319 (-18.8516, -225.0409) -> (-19.2614, -224.9311) centre (-19.1114, -225.1909) ccw
  arc A320 (-16.2303, -223.1811) -> (-16.3401, -223.5909) centre (-16.0803, -223.4409) ccw
  arc A321 (-18.3766, -225.8636) -> (-17.0106, -226.2297) centre (-17.5106, -225.3636) ccw
  arc A322 (-14.9311, -229.2614) -> (-15.0409, -228.8516) centre (-15.1909, -229.1114) ccw
  arc A323 (-14.4636, -225.9518) -> (-15.8297, -226.3178) centre (-14.9636, -226.8178) ccw
  arc A324 (-9.8651, -222.4868) -> (-11.2311, -222.8528) centre (-10.3651, -223.3528) ccw
  arc A325 (-5.5153, -226.1528) -> (-5.8814, -224.7868) centre (-6.3814, -225.6528) ccw
  line L296 (-9.2153, -232.5614) -> (-9.4969, -233.0491)
  line L297 (-15.0409, -228.8516) -> (-15.8636, -228.3766)
  arc A326 (-15.9586, -229.889) -> (-15.2126, -229.7491) centre (-15.6457, -229.4991) ccw
  line L298 (-15.8297, -226.3178) -> (-16.2297, -227.0106)
  line L299 (-13.6409, -226.4268) -> (-14.4636, -225.9518)
  line L300 (-14.9311, -229.2614) -> (-15.2126, -229.7491)
  line L301 (-7.4653, -229.5303) -> (-5.5153, -226.1528)
  arc A327 (-16.2297, -227.0106) -> (-15.8636, -228.3766) centre (-15.3636, -227.5106) ccw
  line L302 (-5.8814, -224.7868) -> (-9.8651, -222.4868)
  arc A328 (-13.6409, -226.4268) -> (-13.2311, -226.3169) centre (-13.4909, -226.1669) ccw
  line L303 (-11.2311, -222.8528) -> (-13.2311, -226.3169)
  arc A329 (-9.4969, -233.0491) -> (-9.2451, -233.765) centre (-9.0639, -233.2991) ccw
  arc A330 (-6.1668, -231.7812) -> (-6.5328, -230.4151) centre (-7.0328, -231.2812) ccw
  line L304 (-8.8055, -232.4516) -> (-7.9828, -232.9266)
  line L305 (-6.6168, -232.5606) -> (-6.1668, -231.7812)
  line L306 (-6.5328, -230.4151) -> (-7.3555, -229.9401)
  arc A331 (-8.8055, -232.4516) -> (-9.2153, -232.5614) centre (-8.9555, -232.7114) ccw
  arc A332 (-7.4653, -229.5303) -> (-7.3555, -229.9401) centre (-7.2055, -229.6803) ccw
  arc A333 (-7.9828, -232.9266) -> (-6.6168, -232.5606) centre (-7.4828, -232.0606) ccw
  arc A334 (3.876, -235.2037) -> (9.2451, -233.765) centre (0, -210) ccw
  arc A335 (15.9586, -229.889) -> (19.889, -225.9586) centre (0, -210) ccw
  arc A336 (23.765, -219.2451) -> (25.2037, -213.876) centre (0, -210) ccw
  arc A337 (25.2037, -206.124) -> (23.765, -200.7549) centre (0, -210) ccw
  arc A338 (19.889, -194.0414) -> (15.9586, -190.111) centre (0, -210) ccw
  arc A339 (9.2451, -186.235) -> (3.876, -184.7963) centre (0, -210) ccw
  arc A340 (-3.876, -184.7963) -> (-9.2451, -186.235) centre (0, -210) ccw
  arc A341 (-15.9586, -190.111) -> (-19.889, -194.0414) centre (0, -210) ccw
  arc A342 (-23.765, -200.7549) -> (-25.2037, -206.124) centre (0, -210) ccw
  arc A343 (-25.2037, -213.876) -> (-23.765, -219.2451) centre (0, -210) ccw
  arc A344 (-19.889, -225.9586) -> (-15.9586, -229.889) centre (0, -210) ccw
  arc A345 (-9.2451, -233.765) -> (-3.876, -235.2037) centre (0, -210) ccw
  line L307 (3.3, -234.1464) -> (3.3, -230.6464)
  line L308 (-3.3, -234.1464) -> (-3.3, -230.7464)
  line L309 (14.9311, -229.2614) -> (13.1811, -226.2303)
  line L310 (9.2153, -232.5614) -> (7.5153, -229.6169)
  line L311 (22.5614, -219.2153) -> (19.5303, -217.4653)
  line L312 (19.2614, -224.9311) -> (16.3169, -223.2311)
  line L313 (24.1464, -206.7) -> (20.6464, -206.7)
  line L314 (24.1464, -213.3) -> (20.7464, -213.3)
  line L315 (19.2614, -195.0689) -> (16.2303, -196.8189)
  line L316 (22.5614, -200.7847) -> (19.6169, -202.4847)
  line L317 (9.2153, -187.4386) -> (7.4653, -190.4697)
  line L318 (14.9311, -190.7386) -> (13.2311, -193.6831)
  line L319 (-3.3, -185.8536) -> (-3.3, -189.3536)
  line L320 (3.3, -185.8536) -> (3.3, -189.2536)
  line L321 (-14.9311, -190.7386) -> (-13.1811, -193.7697)
  line L322 (-9.2153, -187.4386) -> (-7.5153, -190.3831)
  line L323 (-22.5614, -200.7847) -> (-19.5303, -202.5347)
  line L324 (-19.2614, -195.0689) -> (-16.3169, -196.7689)
  line L325 (-24.1464, -213.3) -> (-20.6464, -213.3)
  line L326 (-24.1464, -206.7) -> (-20.7464, -206.7)
  line L327 (-19.2614, -224.9311) -> (-16.2303, -223.1811)
  line L328 (-22.5614, -219.2153) -> (-19.6169, -217.5153)
  line L329 (-9.2153, -232.5614) -> (-7.4653, -229.5303)
  line L330 (-14.9311, -229.2614) -> (-13.2311, -226.3169)
  line L331 (-22.5614, -284.2153) -> (-19.6169, -282.5153)
  line L332 (-22.5614, -284.2153) -> (-23.0491, -284.4969)
  arc A346 (-23.8464, -278.6) -> (-24.1464, -278.3) centre (-24.1464, -278.6) ccw
  arc A347 (-22.5614, -284.2153) -> (-22.4516, -283.8055) centre (-22.7114, -283.9555) ccw
  arc A348 (-20.0267, -282.4055) -> (-19.6169, -282.5153) centre (-19.7669, -282.2555) ccw
  arc A349 (-20.6464, -278.3) -> (-20.9464, -278.6) centre (-20.6464, -278.6) ccw
  line L333 (-21.8678, -281.2168) -> (-22.5606, -281.6168)
  line L334 (-24.1464, -278.3) -> (-24.7095, -278.3)
  arc A350 (-25.2037, -278.876) -> (-23.765, -284.2451) centre (0, -275) ccw
  line L335 (-22.4516, -283.8055) -> (-22.9266, -282.9828)
  arc A351 (-16.7464, -278.3) -> (-15.7464, -277.3) centre (-16.7464, -277.3) ccw
  arc A352 (-24.7095, -278.3) -> (-25.2037, -278.876) centre (-24.7095, -278.8) ccw
  line L336 (-23.8464, -278.6) -> (-23.8464, -279.55)
  line L337 (-20.6464, -278.3) -> (-16.7464, -278.3)
  arc A353 (-12.8528, -286.2311) -> (-12.4868, -284.8651) centre (-13.3528, -285.3651) ccw
  arc A354 (-14.7868, -280.8814) -> (-16.1528, -280.5153) centre (-15.6528, -281.3814) ccw
  arc A355 (-4.55, -296.0464) -> (-5.55, -297.0464) centre (-4.55, -297.0464) ccw
  arc A356 (-6.6168, -252.4394) -> (-7.9828, -252.0734) centre (-7.4828, -252.9394) ccw
  line L338 (-5.5153, -258.8472) -> (-7.5153, -255.3831)
  line L339 (-5.55, -297.0464) -> (-5.55, -297.8464)
  arc A357 (2.3, -259.2536) -> (3.3, -258.2536) centre (2.3, -258.2536) ccw
  arc A358 (-7.9828, -297.9266) -> (-6.6168, -297.5606) centre (-7.4828, -297.0606) ccw
  arc A359 (3.6, -298.8464) -> (3.3, -299.1464) centre (3.6, -299.1464) ccw
  line L340 (-5.55, -252.1536) -> (-5.55, -253.0536)
  arc A360 (-5.55, -253.0536) -> (-4.55, -254.0536) centre (-4.55, -253.0536) ccw
  line L341 (-7.4653, -294.5303) -> (-5.5153, -291.1528)
  line L342 (-3.3, -250.8536) -> (-3.3, -254.3536)
  line L343 (-6.5328, -295.4151) -> (-7.3555, -294.9401)
  arc A361 (3.876, -249.7963) -> (3.3, -250.2905) centre (3.8, -250.2905) ccw
  arc A362 (3.3, -295.6464) -> (3.6, -295.9464) centre (3.6, -295.6464) ccw
  line L344 (-3.6, -296.0464) -> (-4.55, -296.0464)
  line L345 (3.3, -295.6464) -> (3.3, -291.7464)
  arc A363 (-3.3, -299.1464) -> (-3.6, -298.8464) centre (-3.6, -299.1464) ccw
  line L346 (3.3, -299.1464) -> (3.3, -295.6464)
  arc A364 (-3.3, -250.2905) -> (-3.876, -249.7963) centre (-3.8, -250.2905) ccw
  arc A365 (-6.1668, -296.7812) -> (-6.5328, -295.4151) centre (-7.0328, -296.2812) ccw